Autodesk Inventor part; units mm, degrees
(part 14 of 18)
  line L295 (-10.395, -13.6654) -> (-10.3935, -13.6958)
  line L296 (9.9244, -17.7186) -> (9.9274, -17.7184)
  line L297 (10.1429, -17.706) -> (10.2016, -17.7027)
  line L298 (10.0945, -17.6651) -> (10.2016, -17.7027)
  line L299 (10.0388, -17.6683) -> (10.0945, -17.6651)
  line L300 (10.2016, -17.7027) -> (10.2019, -17.698)
  line L301 (10.0945, -17.6651) -> (10.0974, -17.6073)
  line L302 (10.1899, -15.782) -> (10.1905, -15.7701)
  line L303 (10.5029, -17.7271) -> (10.5027, -17.7312)
  line L304 (10.6831, -17.7208) -> (10.5027, -17.7312)
  line L305 (10.684, -17.7017) -> (10.6831, -17.7208)
  line L306 (10.5027, -17.7312) -> (10.9975, -17.9047)
  line L307 (11.1778, -17.8943) -> (10.9975, -17.9047)
  line L308 (10.6831, -17.7208) -> (11.1778, -17.8943)
  line L309 (11.1778, -17.8943) -> (11.1805, -17.8415)
  line L310 (11.0279, -17.9924) -> (10.9208, -17.9548)
  line L311 (11.0304, -17.9434) -> (11.0279, -17.9924)
  line L312 (10.9208, -17.9548) -> (10.6544, -17.9701)
  line L313 (11.0279, -17.9924) -> (10.6522, -18.014)
  line L314 (-10.131, -17.7025) -> (-10.0641, -17.6809)
  line L315 (-10.2521, -17.6674) -> (-10.0641, -17.6809)
  line L316 (-10.3599, -17.7021) -> (-10.2521, -17.6674)
  line L317 (-10.0641, -17.6809) -> (-10.0644, -17.6303)
  line L318 (-10.0765, -15.7777) -> (-10.0792, -15.3552)
  line L319 (-10.2521, -17.6674) -> (-10.2524, -17.6239)
  line L320 (-10.2645, -15.7689) -> (-10.2646, -15.7629)
  line L321 (-10.2782, -13.6655) -> (-10.2784, -13.6388)
  line L322 (9.0029, -17.7241) -> (9.7279, -17.6637)
  line L323 (9.6237, -17.6343) -> (9.7279, -17.6637)
  line L324 (9.3477, -17.6573) -> (9.6237, -17.6343)
  line L325 (9.7279, -17.6637) -> (9.728, -17.6538)
  line L326 (9.6237, -17.6343) -> (9.6238, -17.6121)
  line L327 (9.6503, -13.6367) -> (9.6506, -13.6057)
  line L328 (-7.4275, 0.4913) -> (-8.4227, 0.5954)
  line L329 (-11.2211, 1.3907) -> (-8.3706, 1.0926)
  ellipse E238 centre (-9.068, 1.1652) end of major axis (-11.5544, 1.4256) minor radius 0.0002 (-11.2211, 1.3907) -> (-11.5544, 1.4256) ccw
  line L330 (-11.7521, -0.4624) -> (-11.5544, 1.4256)
  line L331 (8.4338, 0.5941) -> (7.4385, 0.4902)
  line L332 (8.3818, 1.0914) -> (11.2323, 1.389)
  ellipse E239 centre (9.0792, 1.1638) end of major axis (11.5656, 1.4238) minor radius 0.0002 (11.5656, 1.4238) -> (11.2323, 1.389) ccw
  line L333 (11.5656, 1.4238) -> (11.763, -0.4642)
  ellipse E240 centre (-8.7944, -3.3251) end of major axis (-9.0427, -3.2961) minor radius 0
  ellipse E241 centre (-7.7259, -3.45) end of major axis (-8.3188, -3.3807) minor radius 0 (-8.2679, -3.3867) -> (-8.2679, -3.3867) ccw
  ellipse E242 centre (-11.2149, -3.0423) end of major axis (-10.4244, -3.1347) minor radius 0 (-11.5644, -3.0014) -> (-11.5645, -3.0015) ccw
  line L334 (-8.2679, -3.3865) -> (-12.108, -2.9378)
  ellipse E243 centre (-9.9578, -3.1893) end of major axis (-12.4408, -2.899) minor radius 0.0001 (-12.1007, -2.9387) -> (-12.4408, -2.899) ccw
  line L335 (-11.8177, -0.4547) -> (-8.9714, -0.7873)
  ellipse E244 centre (-9.6674, -0.7062) end of major axis (-12.1505, -0.4159) minor radius 0.0001 (-11.8177, -0.4547) -> (-12.1505, -0.4159) ccw
  line L336 (-12.4408, -2.899) -> (-12.1505, -0.4159)
  ellipse E245 centre (-4.296, -3.8511) end of major axis (-12.7385, -2.8641) minor radius 0.0004 (-12.3168, -2.9135) -> (-11.5646, -3.0016) ccw
  line L337 (-8.0358, -1.4) -> (-9.0294, -1.2839)
  ellipse E246 centre (8.8048, -3.3264) end of major axis (8.5565, -3.3554) minor radius 0
  ellipse E247 centre (7.7364, -3.4512) end of major axis (8.3292, -3.382) minor radius 0 (8.2784, -3.3879) -> (8.2784, -3.3879) ccw
  ellipse E248 centre (4.3063, -3.8518) end of major axis (12.749, -2.866) minor radius 0.0004 (11.5752, -3.0033) -> (12.3274, -2.9154) ccw
  ellipse E249 centre (9.9682, -3.1908) end of major axis (12.4514, -2.9009) minor radius 0.0001 (12.3274, -2.9154) -> (12.1186, -2.9397) ccw
  line L338 (12.1186, -2.9397) -> (8.2784, -3.3877)
  line L339 (8.9822, -0.7886) -> (11.8286, -0.4565)
  ellipse E250 centre (9.6783, -0.7077) end of major axis (12.1614, -0.4178) minor radius 0.0001 (12.1614, -0.4178) -> (11.8286, -0.4565) ccw
  line L340 (12.1614, -0.4178) -> (12.4514, -2.9009)
  ellipse E251 centre (11.2254, -3.044) end of major axis (10.4349, -3.1363) minor radius 0 (11.575, -3.0032) -> (11.5749, -3.0032) ccw
  line L341 (9.0402, -1.2853) -> (8.0466, -1.4012)
  line L342 (-6.9274, 2.4067) -> (-7.9232, 2.5012)
  line L343 (-10.7288, 3.2695) -> (-7.876, 2.999)
  ellipse E252 centre (-8.5735, 3.0651) end of major axis (-11.0623, 3.3012) minor radius 0 (-10.7288, 3.2695) -> (-11.0623, 3.3012) ccw
  line L344 (-11.2433, 1.3931) -> (-11.0623, 3.3012)
  line L345 (4.0938, 2.5867) -> (4.0057, 2.6011)
  line L346 (-3.9943, 2.6018) -> (-4.0824, 2.5874)
  line L347 (-5.7789, 2.8081) -> (-4.9943, 2.9362)
  line L348 (5.0057, 2.9355) -> (5.7903, 2.8072)
  line L349 (7.9346, 2.5) -> (6.9387, 2.4057)
  line L350 (7.8874, 2.9978) -> (10.7403, 3.2679)
  ellipse E253 centre (8.5849, 3.0638) end of major axis (11.0738, 3.2995) minor radius 0 (11.0738, 3.2995) -> (10.7403, 3.2679) ccw
  line L351 (11.0738, 3.2995) -> (11.2545, 1.3914)
  spline S0 degree 3 poles (-6.2703, 3.3864) (-6.2254, 3.4062) (-6.1365, 3.4454) (-6.0037, 3.5016) (-5.8729, 3.5551) (-5.7026, 3.622) (-5.494, 3.6996) (-5.3264, 3.7547) (-5.2441, 3.7817) knots 0 0 0 0 0.13379 0.264806 0.393183 0.519054 0.763783 1 1 1 1
  line L352 (-6.3254, 2.8599) -> (-6.2703, 3.3864)
  spline S1 degree 3 poles (-7.398, 3.7442) (-7.4114, 3.7431) (-7.4379, 3.741) (-7.477, 3.7389) (-7.5148, 3.7377) (-7.5511, 3.7377) (-7.5857, 3.7387) (-7.6185, 3.7408) (-7.6494, 3.744) (-7.6783, 3.7482) (-7.7052, 3.7533) (-7.7301, 3.7594) (-7.7528, 3.7663) (-7.7735, 3.774) (-7.7922, 3.7826) (-7.8092, 3.7922) (-7.8246, 3.8026) (-7.8337, 3.8106) (-7.8382, 3.8146) knots 0 0 0 0 0.088475 0.174424 0.25743 0.337089 0.413015 0.484966 0.552919 0.616878 0.676853 0.732867 0.784956 0.833184 0.87778 0.920162 0.960829 1 1 1 1
  ellipse E254 centre (-3.1382, 3.0582) end of major axis (-8.5695, 3.6268) minor radius 0.0004 (-6.2703, 3.3864) -> (-8.5695, 3.6268) ccw
  line L353 (-8.2557, 3.8812) -> (-8.5695, 3.6268)
  line L354 (-8.6278, 3.0703) -> (-8.5695, 3.6268)
  spline S2 degree 3 poles (-3.1442, 3.5227) (-3.1016, 3.547) (-3.0173, 3.5949) (-2.891, 3.6642) (-2.7665, 3.7307) (-2.6041, 3.8145) (-2.4047, 3.9129) (-2.2437, 3.9847) (-2.1647, 4.0199) knots 0 0 0 0 0.133763 0.26476 0.393126 0.518994 0.763738 1 1 1 1
  line L355 (-3.1442, 3.341) -> (-3.1442, 3.5227)
  line L356 (3.1557, 3.5222) -> (3.1557, 3.3405)
  spline S3 degree 3 poles (2.1763, 4.0196) (2.2553, 3.9843) (2.4162, 3.9125) (2.6156, 3.8141) (2.7781, 3.7302) (2.9026, 3.6638) (3.0288, 3.5945) (3.1131, 3.5465) (3.1557, 3.5222) knots 0 0 0 0 0.236262 0.481006 0.606874 0.73524 0.866237 1 1 1 1
  line L357 (-2.1647, 4.0199) -> (2.1763, 4.0196)
  ellipse E255 centre (0.0058, 3.5555) end of major axis (-4.9552, 3.5559) minor radius 0.5163 (2.6804, 3.9901) -> (2.1763, 4.0196) ccw
  ellipse E256 centre (0.0058, 3.5555) end of major axis (-4.9552, 3.5559) minor radius 0.5163 (-2.1647, 4.0199) -> (-2.6688, 3.9905) ccw
  ellipse E257 centre (0.0057, 3.0582) end of major axis (5.4667, 3.0578) minor radius 0.5683 (5.3031, 3.1959) -> (3.1557, 3.5222) ccw
  ellipse E258 centre (0.0057, 3.0582) end of major axis (-5.4553, 3.0586) minor radius 0.5683 (-3.1442, 3.5227) -> (-5.2916, 3.1967) ccw
  line L358 (6.2817, 3.3855) -> (6.3368, 2.859)
  spline S4 degree 3 poles (5.2556, 3.7809) (5.3379, 3.7538) (5.5055, 3.6987) (5.7141, 3.6211) (5.8844, 3.5542) (6.0152, 3.5007) (6.148, 3.4445) (6.2369, 3.4053) (6.2817, 3.3855) knots 0 0 0 0 0.236217 0.480946 0.606817 0.735194 0.86621 1 1 1 1
  spline S5 degree 3 poles (7.8493, 3.8136) (7.8447, 3.8096) (7.8351, 3.8013) (7.8189, 3.7906) (7.8009, 3.7807) (7.7812, 3.7719) (7.7597, 3.7639) (7.7365, 3.757) (7.7115, 3.751) (7.6849, 3.7461) (7.6565, 3.7422) (7.6263, 3.7393) (7.5943, 3.7375) (7.5606, 3.7366) (7.525, 3.7368) (7.4878, 3.738) (7.449, 3.7401) (7.4226, 3.7422) (7.4091, 3.7433) knots 0 0 0 0 0.040391 0.082789 0.1275 0.174786 0.22486 0.277901 0.334055 0.393442 0.45616 0.522411 0.592561 0.666584 0.744418 0.825989 0.911213 1 1 1 1
  ellipse E259 centre (3.1496, 3.0577) end of major axis (8.581, 3.6255) minor radius 0.0004 (8.581, 3.6255) -> (6.2817, 3.3855) ccw
  line L359 (8.2673, 3.8799) -> (8.581, 3.6255)
  line L360 (8.6392, 3.0689) -> (8.581, 3.6255)
  spline S6 degree 3 poles (-5.7981, 5.3131) (-5.7534, 5.3333) (-5.6649, 5.3734) (-5.5327, 5.4308) (-5.4024, 5.4856) (-5.2327, 5.5541) (-5.0249, 5.6338) (-4.8578, 5.6905) (-4.7758, 5.7183) knots 0 0 0 0 0.13379 0.264806 0.393183 0.519054 0.763783 1 1 1 1
  line L361 (-5.9686, 3.5159) -> (-5.7981, 5.3131)
  line L362 (-4.7758, 5.7183) -> (-3.9801, 5.6429)
  ellipse E260 centre (-2.6153, 5.5133) end of major axis (-7.5542, 5.9819) minor radius 0.0001 (-7.3844, 5.9658) -> (-7.5542, 5.9819) ccw
  ellipse E261 centre (-2.6153, 5.5133) end of major axis (-7.5542, 5.9819) minor radius 0.0001 (-4.7758, 5.7183) -> (-6.1112, 5.845) ccw
  spline S7 degree 3 poles (-6.1112, 5.845) (-6.1628, 5.8292) (-6.2638, 5.7981) (-6.4132, 5.7573) (-6.5562, 5.7223) (-6.692, 5.6938) (-6.8208, 5.672) (-6.9424, 5.6575) (-7.0389, 5.6518) (-7.1106, 5.6521) (-7.1588, 5.6549) (-7.2029, 5.66) (-7.2426, 5.6672) (-7.2779, 5.6764) (-7.3174, 5.6905) (-7.3588, 5.7133) (-7.3959, 5.7512) (-7.4169, 5.7986) (-7.4195, 5.8521) (-7.4083, 5.9091) (-7.3926, 5.9463) (-7.3844, 5.9658) knots 0 0 0 0 0.104135 0.203976 0.298889 0.388275 0.471711 0.551067 0.624597 0.658204 0.689291 0.717816 0.743784 0.767218 0.788166 0.824633 0.857384 0.888881 0.922221 0.959245 1 1 1 1
  ellipse E262 centre (-2.6626, 5.0156) end of major axis (-8.0992, 5.5313) minor radius 0.0001 (-5.7981, 5.3131) -> (-8.0992, 5.5313) ccw
  line L363 (-7.5542, 5.9819) -> (-8.0992, 5.5313)
  ellipse E263 centre (-6.0533, 5.8395) end of major axis (-4.5488, 5.6968) minor radius 0 (-7.3848, 5.9658) -> (-6.194, 5.8528) ccw
  line L364 (-8.2557, 3.8812) -> (-8.0992, 5.5313)
  spline S8 degree 3 poles (-3.144, 5.4364) (-3.1014, 5.4606) (-3.0171, 5.5087) (-2.8909, 5.578) (-2.7664, 5.6445) (-2.6039, 5.7284) (-2.4045, 5.8269) (-2.2436, 5.8988) (-2.1645, 5.9341) knots 0 0 0 0 0.133768 0.264768 0.393136 0.519004 0.763746 1 1 1 1
  line L365 (-3.1442, 3.7223) -> (-3.144, 5.4364)
  line L366 (3.1558, 5.4359) -> (3.1557, 3.7218)
  spline S9 degree 3 poles (2.1764, 5.9337) (2.2555, 5.8984) (2.4164, 5.8265) (2.6158, 5.728) (2.7782, 5.6441) (2.9027, 5.5776) (3.0289, 5.5082) (3.1132, 5.4602) (3.1558, 5.4359) knots 0 0 0 0 0.236254 0.480996 0.606864 0.735232 0.866232 1 1 1 1
  line L367 (-2.1645, 5.9341) -> (2.1764, 5.9337)
  ellipse E264 centre (0.0059, 5.5131) end of major axis (-4.9551, 5.5135) minor radius 0.4679 (3.5178, 5.8434) -> (2.1764, 5.9337) ccw
  ellipse E265 centre (0.0059, 5.5131) end of major axis (-4.9551, 5.5135) minor radius 0.4679 (-2.1645, 5.9341) -> (-3.5059, 5.8439) ccw
  spline S10 degree 3 poles (-3.5059, 5.8439) (-3.546, 5.8257) (-3.625, 5.7899) (-3.7424, 5.739) (-3.8563, 5.6915) (-3.9663, 5.6478) (-4.0719, 5.6081) (-4.1733, 5.5723) (-4.2708, 5.5406) (-4.364, 5.5134) (-4.451, 5.4913) (-4.5297, 5.4754) (-4.5985, 5.4659) (-4.6566, 5.4624) (-4.7048, 5.4646) (-4.7435, 5.473) (-4.775, 5.4866) (-4.7885, 5.5022) (-4.7948, 5.5095) knots 0 0 0 0 0.096483 0.190064 0.280343 0.366935 0.449463 0.527566 0.602572 0.674179 0.740358 0.79923 0.84998 0.89243 0.926709 0.955226 0.979191 1 1 1 1
  spline S11 degree 3 poles (4.8066, 5.5087) (4.8005, 5.5017) (4.7872, 5.4864) (4.756, 5.4729) (4.7173, 5.4645) (4.6697, 5.4619) (4.6138, 5.4648) (4.5492, 5.4734) (4.476, 5.4878) (4.3943, 5.5079) (4.3045, 5.5334) (4.2075, 5.5643) (4.1038, 5.6002) (3.9944, 5.6409) (3.88, 5.6861) (3.7198, 5.7525) (3.5992, 5.8067) (3.5178, 5.8434) knots 0 0 0 0 0.020314 0.043937 0.072556 0.107061 0.147904 0.195304 0.249736 0.311344 0.379674 0.454238 0.534533 0.62004 0.710199 0.804177 1 1 1 1
  ellipse E266 centre (0.0059, 5.0153) end of major axis (5.4669, 5.0149) minor radius 0.5151 (5.1609, 5.185) -> (3.1558, 5.4359) ccw
  ellipse E267 centre (0.0059, 5.0153) end of major axis (-5.4551, 5.0158) minor radius 0.5151 (-3.144, 5.4364) -> (-5.1492, 5.1857) ccw
  line L368 (5.8099, 5.3122) -> (5.9801, 3.515)
  spline S12 degree 3 poles (4.7876, 5.7176) (4.8697, 5.6898) (5.0367, 5.633) (5.2446, 5.5533) (5.4142, 5.4848) (5.5445, 5.43) (5.6767, 5.3725) (5.7652, 5.3324) (5.8099, 5.3122) knots 0 0 0 0 0.236217 0.480946 0.606817 0.735194 0.86621 1 1 1 1
  line L369 (3.9919, 5.6422) -> (4.7876, 5.7176)
  ellipse E268 centre (2.6271, 5.5129) end of major axis (-2.3117, 5.0452) minor radius 0.0001 (6.1245, 5.8442) -> (4.7895, 5.7178) ccw
  ellipse E269 centre (2.6271, 5.5129) end of major axis (7.566, 5.9807) minor radius 0.0001 (7.566, 5.9807) -> (7.3962, 5.9646) ccw
  spline S13 degree 3 poles (7.3963, 5.9646) (7.4047, 5.9446) (7.4206, 5.9071) (7.4315, 5.85) (7.4286, 5.7975) (7.4082, 5.7511) (7.3712, 5.7135) (7.3197, 5.6848) (7.2544, 5.6647) (7.1751, 5.6529) (7.0818, 5.6498) (6.9749, 5.6549) (6.8553, 5.668) (6.7244, 5.689) (6.5837, 5.7176) (6.435, 5.7537) (6.2803, 5.7958) (6.176, 5.8278) (6.1231, 5.8441) knots 0 0 0 0 0.041849 0.07857 0.111147 0.141904 0.174268 0.211184 0.254599 0.305659 0.365519 0.434561 0.512207 0.59776 0.690456 0.789354 0.89303 1 1 1 1
  ellipse E270 centre (2.6743, 5.0152) end of major axis (8.111, 5.5301) minor radius 0.0001 (8.111, 5.5301) -> (5.8099, 5.3122) ccw
  line L370 (7.566, 5.9807) -> (8.111, 5.5301)
  line L371 (8.2673, 3.8799) -> (8.111, 5.5301)
  ellipse E271 centre (-2.8258, 6.0418) end of major axis (-6.7195, 6.4495) minor radius 0.0003 (-3.1855, 6.0798) -> (-4.4498, 6.2121) ccw
  ellipse E272 centre (-4.7647, 6.2451) end of major axis (-4.5658, 6.2242) minor radius 0 (-4.6559, 6.2337) -> (-4.5658, 6.2242) ccw
  line L372 (-4.5657, 6.2243) -> (-4.5658, 6.2242)
  ellipse E273 centre (-4.3668, 6.2034) end of major axis (-4.5657, 6.2243) minor radius 0 (-4.4498, 6.2121) -> (-4.5657, 6.2243) ccw
  ellipse E274 centre (-2.8258, 6.0418) end of major axis (-6.1725, 6.3923) minor radius 0.0002 (-4.6559, 6.2337) -> (-6.1725, 6.3923) ccw
  line L373 (-6.1725, 6.3923) -> (-6.2286, 5.8561)
  ellipse E275 centre (-1.1805, 21.7559) end of major axis (-3.4282, 21.9913) minor radius 0.0002 (-3.154, 21.9627) -> (-3.4282, 21.9913) ccw
  line L374 (-3.4282, 21.9913) -> (-3.7247, 20.0442)
  line L375 (1.7559, 5.9338) -> (1.756, 6.3932)
  ellipse E276 centre (1.556, 6.3932) end of major axis (1.756, 6.3932) minor radius 0.0208 (1.756, 6.3932) -> (1.6394, 6.4121) ccw
  ellipse E277 centre (0.0059, 6.0419) end of major axis (-3.9091, 6.0422) minor radius 0.4074 (1.6394, 6.4121) -> (-1.6275, 6.4123) ccw
  ellipse E278 centre (1.956, 6.3524) end of major axis (1.756, 6.3524) minor radius 0.0208 (1.756, 6.3524) -> (1.8466, 6.335) ccw
  ellipse E279 centre (-1.944, 6.3527) end of major axis (-1.744, 6.3526) minor radius 0.0208 (-1.8346, 6.3352) -> (-1.744, 6.3526) ccw
  ellipse E280 centre (-1.544, 6.3934) end of major axis (-1.744, 6.3934) minor radius 0.0208 (-1.6275, 6.4123) -> (-1.744, 6.3934) ccw
  line L376 (-1.744, 6.3934) -> (-1.7441, 5.934)
  ellipse E281 centre (0.0059, 6.0419) end of major axis (3.3709, 6.0417) minor radius 0.3502 (3.3338, 6.0936) -> (1.8466, 6.335) ccw
  ellipse E282 centre (0.0059, 6.0419) end of major axis (-3.3591, 6.0422) minor radius 0.3502 (-1.8346, 6.3352) -> (-3.3219, 6.0941) ccw
  ellipse E283 centre (0.0071, 21.7561) end of major axis (2.2671, 21.756) minor radius 0.2352 (1.0452, 21.965) -> (-1.0309, 21.9651) ccw
  ellipse E284 centre (4.3787, 6.2028) end of major axis (4.5776, 6.2236) minor radius 0 (4.5776, 6.2236) -> (4.4617, 6.2115) ccw
  ellipse E285 centre (2.8377, 6.0414) end of major axis (-1.0561, 5.6343) minor radius 0.0003 (4.4617, 6.2115) -> (3.1974, 6.0793) ccw
  line L377 (4.5777, 6.2235) -> (4.5776, 6.2236)
  ellipse E286 centre (4.7766, 6.2443) end of major axis (4.5777, 6.2235) minor radius 0 (4.5777, 6.2235) -> (4.6678, 6.233) ccw
  ellipse E287 centre (2.8377, 6.0414) end of major axis (6.1844, 6.3913) minor radius 0.0002 (6.1844, 6.3913) -> (4.6678, 6.233) ccw
  line L378 (6.1844, 6.3913) -> (6.2405, 5.8552)
  ellipse E288 centre (1.1948, 21.7558) end of major axis (3.4425, 21.9908) minor radius 0.0002 (3.4425, 21.9908) -> (3.1684, 21.9622) ccw
  line L379 (3.4425, 21.9908) -> (3.7387, 20.0436)
  ellipse E289 centre (-1.5322, 19.7878) end of major axis (-3.7769, 20.0503) minor radius 0.0001 (-3.0188, 19.9617) -> (-3.7769, 20.0503) ccw
  line L380 (-3.7769, 20.0503) -> (-5.7087, 8.318)
  line L381 (-5.7576, 8.0211) -> (-6.0282, 6.3772)
  ellipse E290 centre (0.0058, 4.0949) end of major axis (-3.9092, 4.0952) minor radius 0.4538 (0.7242, 4.541) -> (0.6204, 4.5431) ccw
  ellipse E291 centre (0.0058, 4.0949) end of major axis (-3.9092, 4.0952) minor radius 0.4538 (0.3465, 4.547) -> (-0.3898, 4.5465) ccw
  ellipse E292 centre (0.0058, 4.0949) end of major axis (-3.9092, 4.0952) minor radius 0.4538 (-0.6087, 4.5432) -> (-0.7125, 4.5411) ccw
  ellipse E293 centre (0.007, 19.7884) end of major axis (2.267, 19.7882) minor radius 0.262 (1.716, 19.9597) -> (-1.702, 19.96) ccw
  ellipse E294 centre (1.5462, 19.7876) end of major axis (3.791, 20.0497) minor radius 0.0001 (3.791, 20.0497) -> (3.0328, 19.9613) ccw
  line L382 (3.791, 20.0497) -> (5.7209, 8.3171)
  line L383 (5.7697, 8.0202) -> (6.0402, 6.3763)
  ellipse E295 centre (-0.7937, 24.7162) end of major axis (-0.5896, 24.6969) minor radius 0 (-0.5896, 24.6969) -> (-0.8355, 24.7202) ccw
  ellipse E296 centre (-0.8349, 24.2822) end of major axis (-2.0644, 24.3988) minor radius 0 (-1.1783, 24.3148) -> (-2.0644, 24.3988) ccw
  line L384 (-2.0644, 24.3988) -> (-2.1166, 23.8482)
  arc A0 (-1.1612, 24.7267) -> (-2.0644, 24.3988) centre (-0.9749, 22.8057) ccw
  arc A1 (-0.4838, 24.6722) -> (-0.5896, 24.6969) centre (-0.9749, 22.8057) ccw
  ellipse E297 centre (-2.3792, 8.0022) end of major axis (-6.2767, 8.3719) minor radius 0 (-3.0173, 8.0627) -> (-4.0051, 8.1564) ccw
  ellipse E298 centre (-2.4737, 7.0066) end of major axis (-6.3712, 7.3764) minor radius 0 (-2.7241, 7.0304) -> (-4.0996, 7.1609) ccw
  line L385 (-4.1212, 8.1674) -> (-4.1212, 8.1674)
  line L386 (-4.2156, 7.1719) -> (-4.2156, 7.1719)
  ellipse E299 centre (-2.3792, 8.0022) end of major axis (-5.7292, 8.32) minor radius 0 (-4.2114, 8.176) -> (-5.7292, 8.32) ccw
  ellipse E300 centre (-2.4737, 7.0066) end of major axis (-5.8236, 7.3244) minor radius 0 (-4.3059, 7.1805) -> (-5.5824, 7.3016) ccw
  line L387 (-5.7292, 8.32) -> (-5.7576, 8.0211)
  ellipse E301 centre (-0.8871, 23.7316) end of major axis (-3.137, 23.945) minor radius 0 (-1.972, 23.8345) -> (-3.137, 23.945) ccw
  line L388 (-3.137, 23.945) -> (-3.4153, 21.99)
  ellipse E302 centre (0.0073, 24.2822) end of major axis (1.2423, 24.2821) minor radius 0.1165 (1.193, 24.3147) -> (-1.1783, 24.3149) ccw
  arc A2 (-0.1968, 24.7249) -> (-0.9743, 24.4674) centre (0.0072, 22.8057) ccw
  arc A3 (0.989, 24.4673) -> (0.2115, 24.7248) centre (0.0072, 22.8057) ccw
  ellipse E303 centre (1.556, 7.3248) end of major axis (1.756, 7.3248) minor radius 0.0189 (1.756, 7.3248) -> (1.6395, 7.3419) ccw
  line L389 (1.756, 7.3248) -> (1.7561, 8.3203)
  ellipse E304 centre (1.5561, 8.3203) end of major axis (1.7561, 8.3203) minor radius 0.0189 (1.7561, 8.3203) -> (1.6396, 8.3375) ccw
  ellipse E305 centre (0.0061, 8.002) end of major axis (-3.9089, 8.0023) minor radius 0.3693 (1.6396, 8.3375) -> (-1.6273, 8.3377) ccw
  ellipse E306 centre (0.006, 7.0064) end of major axis (-3.909, 7.0067) minor radius 0.3693 (1.6395, 7.3419) -> (-1.6274, 7.3422) ccw
  ellipse E307 centre (1.9561, 8.2833) end of major axis (1.7561, 8.2833) minor radius 0.0189 (1.7561, 8.2833) -> (1.8467, 8.2675) ccw
  ellipse E308 centre (-1.9439, 8.2836) end of major axis (-1.7439, 8.2836) minor radius 0.0189 (-1.8345, 8.2678) -> (-1.7439, 8.2836) ccw
  ellipse E309 centre (-1.5439, 8.3206) end of major axis (-1.7439, 8.3206) minor radius 0.0189 (-1.6273, 8.3377) -> (-1.7439, 8.3206) ccw
  ellipse E310 centre (-1.544, 7.325) end of major axis (-1.744, 7.325) minor radius 0.0189 (-1.6274, 7.3422) -> (-1.744, 7.325) ccw
  line L390 (-1.7439, 8.3206) -> (-1.744, 7.325)
  ellipse E311 centre (1.956, 7.2878) end of major axis (1.756, 7.2878) minor radius 0.0189 (1.756, 7.2878) -> (1.8466, 7.272) ccw
  line L391 (1.756, 7.2878) -> (1.756, 7.3248)
  ellipse E312 centre (-1.944, 7.2881) end of major axis (-1.744, 7.2881) minor radius 0.0189 (-1.8346, 7.2723) -> (-1.744, 7.2881) ccw
  line L392 (-1.744, 7.325) -> (-1.744, 7.2881)
  ellipse E313 centre (0.0061, 8.002) end of major axis (3.3711, 8.0017) minor radius 0.3174 (3.2567, 8.0838) -> (1.8467, 8.2675) ccw
  ellipse E314 centre (0.0061, 8.002) end of major axis (-3.3589, 8.0022) minor radius 0.3174 (-1.8345, 8.2678) -> (-3.2445, 8.0843) ccw
  ellipse E315 centre (0.006, 7.0064) end of major axis (-3.359, 7.0067) minor radius 0.3174 (-3.2638, 7.0816) -> (-3.3332, 7.0459) ccw
  ellipse E316 centre (0.006, 7.0064) end of major axis (3.371, 7.0062) minor radius 0.3174 (-1.8346, 7.2723) -> (-3.0548, 7.1385) ccw
  ellipse E317 centre (0.006, 7.0064) end of major axis (3.371, 7.0062) minor radius 0.3174 (3.0669, 7.1381) -> (1.8466, 7.272) ccw
  ellipse E318 centre (0.006, 7.0064) end of major axis (3.371, 7.0062) minor radius 0.3174 (3.3453, 7.0454) -> (3.2759, 7.0811) ccw
  ellipse E319 centre (0.0073, 23.7315) end of major axis (2.2673, 23.7314) minor radius 0.2132 (1.9869, 23.8342) -> (-1.9723, 23.8345) ccw
  ellipse E320 centre (0.8084, 24.7161) end of major axis (0.6043, 24.6968) minor radius 0 (0.8502, 24.7201) -> (0.6043, 24.6968) ccw
  ellipse E321 centre (0.8495, 24.2821) end of major axis (2.079, 24.3985) minor radius 0 (2.079, 24.3985) -> (1.193, 24.3146) ccw
  line L393 (2.079, 24.3985) -> (2.1312, 23.8479)
  arc A4 (0.6043, 24.6968) -> (0.4985, 24.6721) centre (0.9894, 22.8056) ccw
  arc A5 (2.079, 24.3985) -> (1.1759, 24.7265) centre (0.9894, 22.8056) ccw
  ellipse E322 centre (2.3914, 8.0018) end of major axis (-1.5061, 7.6327) minor radius 0 (4.0179, 8.1559) -> (3.0301, 8.0623) ccw
  ellipse E323 centre (2.4857, 7.0063) end of major axis (-1.4118, 6.6371) minor radius 0 (4.1121, 7.1603) -> (2.7367, 7.0301) ccw
  line L394 (4.1334, 8.1668) -> (4.1334, 8.1668)
  line L395 (4.2277, 7.1713) -> (4.2277, 7.1713)
  ellipse E324 centre (2.3914, 8.0018) end of major axis (5.7414, 8.3191) minor radius 0 (5.7414, 8.3191) -> (4.2235, 8.1754) ccw
  ellipse E325 centre (2.4857, 7.0063) end of major axis (5.8357, 7.3235) minor radius 0 (5.5945, 7.3007) -> (4.3179, 7.1798) ccw
  line L396 (5.7414, 8.3191) -> (5.7697, 8.0202)
  ellipse E326 centre (0.9017, 23.7314) end of major axis (3.1516, 23.9445) minor radius 0 (3.1516, 23.9445) -> (1.9866, 23.8342) ccw
  line L397 (3.1516, 23.9445) -> (3.4296, 21.9894)
  line L398 (7.1686, -28.47) -> (6.503, -26.7548)
  line L399 (9.2433, -28.4702) -> (8.7012, -26.5895)
  line L400 (-9.7907, -28.4687) -> (-9.8927, -26.4495)
  line L401 (-7.7204, -28.4689) -> (-7.6178, -26.5179)
  line L402 (7.1241, -27.8075) -> (6.891, -26.7073)
  line L403 (9.2552, -27.754) -> (9.1137, -26.4991)
  line L404 (-9.2484, -27.7526) -> (-9.1068, -26.4977)
  line L405 (-7.1174, -27.8064) -> (-6.8841, -26.7063)
  line L406 (7.7271, -28.47) -> (7.6247, -26.5191)
  line L407 (9.7974, -28.4702) -> (9.8986, -26.4701)
  line L408 (-9.2366, -28.4688) -> (-8.692, -26.5804)
  line L409 (-7.1619, -28.4689) -> (-6.4961, -26.7538)
  line L410 (7.4032, -27.0593) -> (7.3205, -26.6137)
  line L411 (9.5891, -27.074) -> (9.5284, -26.4528)
  line L412 (-9.5822, -27.0726) -> (-9.5215, -26.4513)
  line L413 (-7.3963, -27.0582) -> (-7.3136, -26.6126)
  ellipse E327 centre (-10.4185, -13.2181) end of major axis (-10.4918, -13.0429) minor radius 0.1721 (-10.5933, -13.21) -> (-10.4874, -13.3848) ccw
  ellipse E328 centre (-10.4771, -13.2427) end of major axis (-10.4038, -13.418) minor radius 0.1721 (-10.6124, -13.3509) -> (-10.5542, -13.4047) ccw
  ellipse E329 centre (-10.4073, -16.022) end of major axis (-10.4807, -15.8468) minor radius 0.1721 (-10.5195, -15.8702) -> (-10.5397, -15.8899) ccw
  ellipse E330 centre (-10.6685, -13.241) end of major axis (-10.6774, -13.4308) minor radius 0.074 (-10.6638, -13.4283) -> (-10.5942, -13.2099) ccw
  ellipse E331 centre (-10.8065, -13.2346) end of major axis (-10.8154, -13.4244) minor radius 0.074 (-10.8018, -13.4218) -> (-10.7322, -13.2035) ccw
  ellipse E332 centre (-10.7367, -16.0139) end of major axis (-10.7278, -15.8241) minor radius 0.074 (-10.6624, -15.9828) -> (-10.7414, -15.8266) ccw
  ellipse E333 centre (-10.3486, -15.9975) end of major axis (-10.422, -15.8222) minor radius 0.1721 (-10.4528, -15.8394) -> (-10.5234, -15.9893) ccw
  ellipse E334 centre (-10.5987, -16.0203) end of major axis (-10.5898, -15.8306) minor radius 0.074 (-10.5244, -15.9893) -> (-10.5898, -15.8306) ccw
  line L414 (-10.5898, -15.8306) -> (-10.7278, -15.8241)
  line L415 (-10.3145, -13.4373) -> (-10.4056, -13.4331)
  line L416 (-10.3317, -13.4092) -> (-10.2128, -13.4148)
  line L417 (-9.7276, -15.6797) -> (-9.7385, -15.2452)
  line L418 (-9.7737, -13.8461) -> (-9.7786, -13.6495)
  line L419 (-11.0395, -13.5213) -> (-10.8018, -13.4218)
  line L420 (-10.6638, -13.4283) -> (-10.7944, -13.483)
  line L421 (-10.7414, -15.8266) -> (-10.842, -15.8687)
  line L422 (-11.0628, -15.7719) -> (-11.1138, -13.7417)
  line L423 (-10.1457, -15.8199) -> (-10.2272, -15.8161)
  line L424 (-10.9758, -13.7481) -> (-10.9248, -15.7784)
  line L425 (-9.7199, -13.6249) -> (-9.7141, -13.8596)
  line L426 (-9.6882, -14.8878) -> (-9.6689, -15.6552)
  ellipse E335 centre (-10.5118, -11.8629) end of major axis (-10.5851, -11.6876) minor radius 0.1721 (-10.5851, -11.6876) -> (-10.6442, -11.7307) ccw
  ellipse E336 centre (-10.3726, -17.4018) end of major axis (-10.2993, -17.5771) minor radius 0.1721 (-10.508, -17.51) -> (-10.4962, -17.5248) ccw
  ellipse E337 centre (-10.314, -17.3773) end of major axis (-10.3873, -17.202) minor radius 0.1721 (-10.4888, -17.3691) -> (-10.4293, -17.5091) ccw
  ellipse E338 centre (-10.4531, -11.8383) end of major axis (-10.5265, -11.6631) minor radius 0.1721 (-10.5117, -11.6577) -> (-10.6279, -11.8302) ccw
  line L427 (-10.5851, -11.6876) -> (-10.5265, -11.6631)
  line L428 (-10.3462, -17.5901) -> (-9.333, -17.6375)
  line L429 (-10.4888, -17.3691) -> (-10.5234, -15.9893)
  line L430 (-9.9216, -17.5827) -> (-10.2724, -17.5663)
  line L431 (-10.244, -11.6611) -> (-10.1954, -11.6634)
  line L432 (-10.5933, -13.21) -> (-10.6279, -11.8302)
  ellipse E339 centre (-9.9024, -15.6716) end of major axis (-9.8291, -15.8468) minor radius 0.1721 (-9.7624, -15.7942) -> (-9.7276, -15.6797) ccw
  ellipse E340 centre (-9.9534, -13.6413) end of major axis (-9.8801, -13.8165) minor radius 0.1721 (-9.7786, -13.6495) -> (-9.7866, -13.5977) ccw
  ellipse E341 centre (-10.9885, -15.7408) end of major axis (-10.9974, -15.9306) minor radius 0.074 (-11.0628, -15.7719) -> (-11.0467, -15.8737) ccw
  ellipse E342 centre (-11.0395, -13.7106) end of major axis (-11.0307, -13.5208) minor radius 0.074 (-11.0571, -13.5316) -> (-11.1138, -13.7417) ccw
  ellipse E343 centre (-9.8948, -13.6167) end of major axis (-9.9681, -13.4415) minor radius 0.1721 (-9.7199, -13.6249) -> (-9.748, -13.5262) ccw
  ellipse E344 centre (-9.8438, -15.647) end of major axis (-9.7704, -15.8223) minor radius 0.1721 (-9.7286, -15.7964) -> (-9.6689, -15.6552) ccw
  ellipse E345 centre (-10.8505, -15.7473) end of major axis (-10.8417, -15.5575) minor radius 0.074 (-10.9248, -15.7784) -> (-10.9147, -15.8595) ccw
  ellipse E346 centre (-10.9015, -13.717) end of major axis (-10.8927, -13.5272) minor radius 0.074 (-10.9721, -13.6754) -> (-10.9758, -13.7481) ccw
  line L433 (-10.7322, -13.2035) -> (-10.7669, -11.8237)
  line L434 (-10.8459, -11.6675) -> (-11.0308, -11.7449)
  line L435 (-11.1442, -17.768) -> (-10.6973, -17.581)
  line L436 (-10.6277, -17.3626) -> (-10.6624, -15.9828)
  line L437 (-10.5942, -13.2099) -> (-10.6289, -11.8301)
  line L438 (-10.4897, -17.3691) -> (-10.5244, -15.9893)
  line L439 (-11.4118, -17.9442) -> (-10.5593, -17.5874)
  ellipse E347 centre (-10.8412, -11.8548) end of major axis (-10.8323, -11.665) minor radius 0.074 (-10.7669, -11.8237) -> (-10.8459, -11.6675) ccw
  ellipse E348 centre (-10.702, -17.3937) end of major axis (-10.7109, -17.5835) minor radius 0.074 (-10.6973, -17.581) -> (-10.6277, -17.3626) ccw
  ellipse E349 centre (-10.7032, -11.8612) end of major axis (-10.6943, -11.6714) minor radius 0.074 (-10.6289, -11.8301) -> (-10.6943, -11.6714) ccw
  ellipse E350 centre (-10.564, -17.4002) end of major axis (-10.5729, -17.5899) minor radius 0.074 (-10.5593, -17.5874) -> (-10.4897, -17.3691) ccw
  line L440 (-10.8323, -11.665) -> (-10.6943, -11.6714)
  line L441 (-10.6433, -18.0256) -> (-11.2796, -17.9959)
  line L442 (-11.3382, -18.0204) -> (-10.6419, -18.053)
  ellipse E351 centre (-11.1818, -17.955) end of major axis (-11.4317, -17.9612) minor radius 0.0419 (-11.4118, -17.9442) -> (-11.2796, -17.9959) ccw
  ellipse E352 centre (-11.1818, -17.955) end of major axis (-11.5817, -17.965) minor radius 0.067 (-11.5798, -17.9582) -> (-11.3382, -18.0204) ccw
  line L443 (-11.5818, -17.9591) -> (-11.5817, -17.965)
  line L444 (9.4455, -13.3827) -> (9.7264, -13.3723)
  line L445 (9.5775, -15.6222) -> (9.4446, -14.3526)
  ellipse E353 centre (9.6129, -11.7904) end of major axis (9.588, -11.6021) minor radius 0.1017 (9.6923, -11.695) -> (9.5932, -11.6016) ccw
  line L446 (9.5932, -11.6016) -> (9.4899, -11.6055)
  line L447 (9.6809, -17.5835) -> (9.9756, -17.5725)
  line L448 (9.9861, -17.5722) -> (10.0546, -17.5696)
  line L449 (9.4941, -17.6023) -> (9.6004, -17.5984)
  ellipse E354 centre (9.6794, -15.6184) end of major axis (9.7043, -15.8068) minor radius 0.1017 (9.5775, -15.6222) -> (9.667, -15.7993) ccw
  ellipse E355 centre (9.4652, -13.5715) end of major axis (9.4404, -13.3831) minor radius 0.1017 (9.4455, -13.3827) -> (9.4451, -13.3827) ccw
  line L450 (-9.3696, -11.6205) -> (-9.4596, -11.6203)
  line L451 (-9.7048, -17.5828) -> (-9.6652, -17.5829)
  line L452 (-9.4762, -17.5832) -> (-9.2454, -17.5836)
  line L453 (-9.1525, -17.3949) -> (-9.0798, -16.7016)
  line L454 (-9.5815, -17.5997) -> (-9.5124, -17.5998)
  ellipse E356 centre (-9.2256, -17.3948) end of major axis (-9.2487, -17.5834) minor radius 0.0727 (-9.2454, -17.5836) -> (-9.1525, -17.3949) ccw
  line L455 (-9.2142, -15.8146) -> (-9.2578, -15.8146)
  ellipse E357 centre (-9.0928, -11.6653) end of major axis (-9.4906, -11.6236) minor radius 0.0171 (-9.4596, -11.6203) -> (-9.4906, -11.6236) ccw
  line L456 (-9.4906, -11.6236) -> (-9.4911, -11.6285)
  line L457 (11.4179, -17.9448) -> (11.0286, -17.9774)
  line L458 (10.6509, -18.039) -> (11.4993, -17.9679)
  ellipse E358 centre (11.4226, -17.7575) end of major axis (11.3708, -17.9403) minor radius 0.1568 (11.4179, -17.9448) -> (11.5023, -17.9099) ccw
  ellipse E359 centre (11.5041, -17.7806) end of major axis (11.4523, -17.9634) minor radius 0.1568 (11.4993, -17.9679) -> (11.5861, -17.9311) ccw
  line L459 (10.6787, -11.6745) -> (10.6474, -11.6656)
  line L460 (10.4979, -17.5791) -> (10.9377, -17.7037)
  line L461 (10.4903, -17.6232) -> (11.5564, -17.9252)
  line L462 (10.603, -13.42) -> (10.9181, -13.5092)
  line L463 (11.0166, -13.7257) -> (10.9653, -15.756)
  ellipse E360 centre (10.2674, -13.4481) end of major axis (10.6672, -13.4582) minor radius 0.067 (10.603, -13.42) -> (10.3781, -13.3865) ccw
  line L464 (9.6449, -13.4205) -> (9.9853, -13.392)
  ellipse E361 centre (10.2674, -13.4481) end of major axis (10.0174, -13.4418) minor radius 0.0419 (10.2515, -13.406) -> (10.1375, -13.4092) ccw
  line L465 (10.6336, -13.4749) -> (10.5682, -13.4563)
  ellipse E362 centre (10.2066, -15.8529) end of major axis (9.8067, -15.8428) minor radius 0.067 (10.5324, -15.8221) -> (10.2569, -15.7877) ccw
  line L466 (9.5478, -13.6455) -> (9.5414, -13.8989)
  ellipse E363 centre (10.9134, -13.6965) end of major axis (10.8975, -13.5072) minor radius 0.1025 (11.0166, -13.7257) -> (10.9181, -13.5092) ccw
  ellipse E364 centre (10.8621, -15.7268) end of major axis (10.8462, -15.5374) minor radius 0.1025 (10.9374, -15.8709) -> (10.9653, -15.756) ccw
  ellipse E365 centre (9.7072, -13.6321) end of major axis (9.759, -13.4493) minor radius 0.1568 (9.559, -13.5808) -> (9.5478, -13.6455) ccw
  ellipse E366 centre (9.6257, -13.609) end of major axis (9.5739, -13.7918) minor radius 0.1568 (9.5907, -13.431) -> (9.4934, -13.5204) ccw
  line L467 (9.3392, -17.6264) -> (9.6361, -17.6015)
  line L468 (9.9681, -17.5737) -> (10.0264, -17.5688)
  ellipse E367 centre (10.1622, -17.6072) end of major axis (10.4122, -17.6136) minor radius 0.0419 (10.1714, -17.5656) -> (10.0264, -17.5688) ccw
  ellipse E368 centre (10.3117, -11.6938) end of major axis (9.9118, -11.6837) minor radius 0.067 (10.6474, -11.6656) -> (10.3438, -11.6278) ccw
  ellipse E369 centre (10.1622, -17.6072) end of major axis (9.7624, -17.5971) minor radius 0.067 (10.4979, -17.5791) -> (10.3333, -17.5509) ccw
  ellipse E370 centre (11.5611, -17.7379) end of major axis (11.577, -17.9273) minor radius 0.1025 (11.5564, -17.9252) -> (11.5756, -17.9274) ccw
  line L469 (9.0712, -17.9822) -> (9.0269, -17.9697)
  ellipse E371 centre (-10.7565, -13.2512) end of major axis (-10.8325, -13.077) minor radius 0.169 (-10.9287, -13.2453) -> (-10.8385, -13.4073) ccw
  ellipse E372 centre (-10.8193, -13.2786) end of major axis (-10.7433, -13.4527) minor radius 0.169 (-10.9475, -13.3912) -> (-10.897, -13.4376) ccw
  ellipse E373 centre (-11.0092, -13.28) end of major axis (-11.0157, -13.4699) minor radius 0.0799 (-10.9998, -13.4667) -> (-10.9296, -13.2453) ccw
  ellipse E374 centre (-11.1452, -13.2754) end of major axis (-11.1517, -13.4653) minor radius 0.0799 (-11.1358, -13.4621) -> (-11.0656, -13.2407) ccw
  ellipse E375 centre (-11.0053, -16.0465) end of major axis (-10.9989, -15.8566) minor radius 0.0799 (-10.9258, -16.0117) -> (-11.0148, -15.8598) ccw
  ellipse E376 centre (-10.6166, -16.0222) end of major axis (-10.6926, -15.8481) minor radius 0.169 (-10.7548, -15.898) -> (-10.7889, -16.0164) ccw
  ellipse E377 centre (-10.8693, -16.0511) end of major axis (-10.8629, -15.8612) minor radius 0.0799 (-10.7898, -16.0164) -> (-10.8629, -15.8612) ccw
  line L470 (-10.8629, -15.8612) -> (-10.9989, -15.8566)
  line L471 (-10.6797, -13.4697) -> (-10.7566, -13.4671)
  line L472 (-10.6912, -13.4398) -> (-10.6159, -13.4423)
  line L473 (-10.0192, -15.6993) -> (-10.0372, -15.3416)
  line L474 (-10.1117, -13.867) -> (-10.1213, -13.675)
  line L475 (-11.3955, -13.5755) -> (-11.1358, -13.4621)
  line L476 (-10.9998, -13.4667) -> (-11.2595, -13.5802)
  line L477 (-12.049, -13.8609) -> (-11.806, -13.7548)
  line L478 (-11.717, -13.9068) -> (-11.6148, -15.931)
  line L479 (-11.685, -16.1525) -> (-11.9279, -16.2586)
  line L480 (-11.0148, -15.8598) -> (-11.2745, -15.9732)
  line L481 (-11.3635, -15.8213) -> (-11.4657, -13.797)
  line L482 (-10.5408, -15.8384) -> (-10.5717, -15.8374)
  line L483 (-11.3297, -13.8016) -> (-11.2275, -15.8259)
  ellipse E378 centre (-11.6863, -13.8732) end of major axis (-12.0858, -13.8934) minor radius 0.0715 (-12.049, -13.8609) -> (-11.8538, -13.9464) ccw
  line L484 (-11.7148, -13.9511) -> (-11.8538, -13.9464)
  line L485 (-11.791, -13.9189) -> (-11.7333, -13.9209)
  ellipse E379 centre (-11.6863, -13.8732) end of major axis (-11.936, -13.8858) minor radius 0.0447 (-11.913, -13.8655) -> (-11.791, -13.9189) ccw
  line L486 (-11.7434, -13.7915) -> (-11.913, -13.8655)
  ellipse E380 centre (-11.5652, -16.2709) end of major axis (-11.9647, -16.291) minor radius 0.0715 (-11.9279, -16.2586) -> (-11.9647, -16.291) ccw
  line L487 (-10.0585, -13.6476) -> (-10.0442, -13.9309)
  line L488 (-9.974, -15.3212) -> (-9.9563, -15.6719)
  ellipse E381 centre (-10.8887, -11.9029) end of major axis (-10.9648, -11.7288) minor radius 0.169 (-10.9648, -11.7288) -> (-11.0189, -11.7687) ccw
  ellipse E382 centre (-10.61, -17.4254) end of major axis (-10.5339, -17.5995) minor radius 0.169 (-10.6154, -17.6109) -> (-10.6005, -17.6121) ccw
  ellipse E383 centre (-10.5471, -17.3979) end of major axis (-10.6232, -17.2238) minor radius 0.169 (-10.5521, -17.5835) -> (-10.5377, -17.5846) ccw
  ellipse E384 centre (-10.5471, -17.3979) end of major axis (-10.6232, -17.2238) minor radius 0.169 (-10.7194, -17.3921) -> (-10.7022, -17.4651) ccw
  ellipse E385 centre (-10.8259, -11.8755) end of major axis (-10.9019, -11.7013) minor radius 0.169 (-10.8958, -11.6988) -> (-10.9982, -11.8696) ccw
  line L489 (-10.9648, -11.7288) -> (-10.9019, -11.7013)
  line L490 (-10.6005, -17.6121) -> (-10.5839, -17.6126)
  line L491 (-10.432, -17.6178) -> (-9.3384, -17.6549)
  line L492 (-10.7194, -17.3921) -> (-10.7889, -16.0164)
  line L493 (-10.2665, -17.5938) -> (-10.3491, -17.591)
  line L494 (-10.5172, -17.5853) -> (-10.5377, -17.5846)
  line L495 (-10.661, -11.6947) -> (-10.6431, -11.6953)
  line L496 (-10.9287, -13.2453) -> (-10.9982, -11.8696)
  ellipse E386 centre (-10.1914, -15.6934) end of major axis (-10.1154, -15.8676) minor radius 0.169 (-10.0321, -15.7797) -> (-10.0192, -15.6993) ccw
  ellipse E387 centre (-10.2936, -13.6692) end of major axis (-10.2176, -13.8433) minor radius 0.169 (-10.1213, -13.675) -> (-10.1287, -13.6298) ccw
  ellipse E388 centre (-11.7966, -13.9415) end of major axis (-11.7901, -13.7516) minor radius 0.0799 (-11.717, -13.9068) -> (-11.806, -13.7548) ccw
  ellipse E389 centre (-11.6944, -15.9658) end of major axis (-11.7008, -16.1557) minor radius 0.0799 (-11.685, -16.1525) -> (-11.6148, -15.931) ccw
  ellipse E390 centre (-11.2839, -15.7865) end of major axis (-11.2903, -15.9764) minor radius 0.0799 (-11.3635, -15.8213) -> (-11.2745, -15.9732) ccw
  ellipse E391 centre (-11.3861, -13.7623) end of major axis (-11.3796, -13.5724) minor radius 0.0799 (-11.3955, -13.5755) -> (-11.4657, -13.797) ccw
  ellipse E392 centre (-10.2308, -13.6418) end of major axis (-10.3068, -13.4676) minor radius 0.169 (-10.0585, -13.6476) -> (-10.0644, -13.6081) ccw
  ellipse E393 centre (-10.1286, -15.666) end of major axis (-10.2046, -15.4919) minor radius 0.169 (-9.9907, -15.7907) -> (-9.9563, -15.6719) ccw
  ellipse E394 centre (-11.1479, -15.7911) end of major axis (-11.1415, -15.6012) minor radius 0.0799 (-11.2275, -15.8259) -> (-11.2011, -15.9412) ccw
  ellipse E395 centre (-11.2501, -13.7669) end of major axis (-11.2436, -13.577) minor radius 0.0799 (-11.2595, -13.5802) -> (-11.3297, -13.8016) ccw
  line L497 (-11.0656, -13.2407) -> (-11.1351, -11.865)
  line L498 (-11.2241, -11.713) -> (-12.1373, -12.1118)
  line L499 (-11.8396, -18.0077) -> (-10.9265, -17.6089)
  line L500 (-10.8563, -17.3875) -> (-10.9258, -16.0117)
  line L501 (-10.9296, -13.2453) -> (-10.9991, -11.8696)
  line L502 (-10.7203, -17.3921) -> (-10.7898, -16.0164)
  line L503 (-11.7036, -18.0123) -> (-10.7905, -17.6135)
  ellipse E396 centre (-11.2147, -11.8997) end of major axis (-11.2082, -11.7098) minor radius 0.0799 (-11.1351, -11.865) -> (-11.2241, -11.713) ccw
  ellipse E397 centre (-10.9359, -17.4222) end of major axis (-10.9423, -17.6121) minor radius 0.0799 (-10.9265, -17.6089) -> (-10.8563, -17.3875) ccw
  ellipse E398 centre (-11.0787, -11.9043) end of major axis (-11.0722, -11.7144) minor radius 0.0799 (-10.9991, -11.8696) -> (-11.0722, -11.7144) ccw
  ellipse E399 centre (-10.7999, -17.4268) end of major axis (-10.8063, -17.6167) minor radius 0.0799 (-10.7905, -17.6135) -> (-10.7203, -17.3921) ccw
  line L504 (-11.2082, -11.7098) -> (-11.0722, -11.7144)
  line L505 (-10.6397, -18.0976) -> (-11.5817, -18.0657)
  line L506 (-11.6445, -18.0931) -> (-10.6382, -18.1273)
  ellipse E400 centre (-11.4769, -18.02) end of major axis (-11.7266, -18.0326) minor radius 0.0447 (-11.7036, -18.0123) -> (-11.5817, -18.0657) ccw
  ellipse E401 centre (-11.7746, -12.1241) end of major axis (-12.1741, -12.1443) minor radius 0.0715 (-12.1373, -12.1118) -> (-12.1741, -12.1443) ccw
  ellipse E402 centre (-11.4769, -18.02) end of major axis (-11.8764, -18.0401) minor radius 0.0715 (-11.8396, -18.0077) -> (-11.6445, -18.0931) ccw
  line L507 (-12.1741, -12.1443) -> (-12.0858, -13.8934)
  line L508 (-11.9647, -16.291) -> (-11.8764, -18.0401)
  ellipse E403 centre (9.6218, -13.1675) end of major axis (9.6454, -13.356) minor radius 0.0959 (9.643, -13.3563) -> (9.7175, -13.1602) ccw
  line L509 (9.6454, -13.356) -> (9.6188, -13.3594)
  line L510 (9.4438, -13.3714) -> (9.643, -13.3563)
  line L511 (9.7998, -15.7892) -> (9.6038, -15.8041)
  line L512 (9.4868, -15.6226) -> (9.3867, -14.7345)
  line L513 (9.7175, -13.1602) -> (9.5608, -11.7693)
  line L514 (9.4437, -11.5879) -> (9.2374, -11.6035)
  line L515 (9.017, -17.6322) -> (9.9579, -17.5607)
  line L516 (8.9456, -17.644) -> (9.5765, -17.5961)
  ellipse E404 centre (9.465, -11.7766) end of major axis (9.4414, -11.5881) minor radius 0.0959 (9.5608, -11.7693) -> (9.4437, -11.5879) ccw
  ellipse E405 centre (9.5825, -15.6153) end of major axis (9.6062, -15.8039) minor radius 0.0959 (9.4868, -15.6226) -> (9.6038, -15.8041) ccw
  ellipse E406 centre (8.6745, -17.6752) end of major axis (8.277, -17.72) minor radius 0.0085 (9.017, -17.6322) -> (8.9464, -17.6383) ccw
  line L517 (-9.2286, -11.6057) -> (-9.3312, -11.599)
  line L518 (-9.8559, -17.5695) -> (-9.1037, -17.6189)
  line L519 (-9.0039, -17.4353) -> (-8.9889, -17.3021)
  line L520 (-9.5406, -17.5979) -> (-8.9681, -17.6355)
  line L521 (-9.5308, -13.3674) -> (-9.4353, -13.3736)
  line L522 (-9.3703, -14.7838) -> (-9.4651, -15.6235)
  line L523 (-9.5648, -15.8072) -> (-9.8044, -15.7914)
  ellipse E407 centre (-9.1693, -13.4117) end of major axis (-9.5667, -13.3669) minor radius 0.0085 (-9.5308, -13.3674) -> (-9.5579, -13.3661) ccw
  ellipse E408 centre (-9.4428, -15.8358) end of major axis (-9.8403, -15.7909) minor radius 0.0085 (-9.8044, -15.7914) -> (-9.8403, -15.7909) ccw
  ellipse E409 centre (-9.5435, -15.6184) end of major axis (-9.5667, -15.807) minor radius 0.0785 (-9.5648, -15.8072) -> (-9.4651, -15.6235) ccw
  ellipse E410 centre (-9.0824, -17.4301) end of major axis (-9.1055, -17.6187) minor radius 0.0785 (-9.1037, -17.6189) -> (-9.0039, -17.4353) ccw
  ellipse E411 centre (-8.9468, -17.4467) end of major axis (-8.9699, -17.6353) minor radius 0.0785 (-8.9681, -17.6355) -> (-8.9398, -17.6258) ccw
  ellipse E412 centre (-8.9697, -11.6434) end of major axis (-9.3672, -11.5985) minor radius 0.0085 (-9.3312, -11.599) -> (-9.3672, -11.5985) ccw
  line L524 (-9.3672, -11.5985) -> (-9.3703, -11.6261)
  line L525 (-9.8403, -15.7909) -> (-9.8415, -15.8014)
  ellipse E413 centre (11.975, -13.724) end of major axis (11.9121, -13.9033) minor radius 0.1599 (11.9656, -13.9107) -> (12.0631, -13.8697) ccw
  ellipse E414 centre (11.8985, -13.6972) end of major axis (11.8356, -13.8765) minor radius 0.1599 (11.8891, -13.8839) -> (11.9795, -13.8486) ccw
  ellipse E415 centre (12.0421, -13.6806) end of major axis (12.053, -13.8703) minor radius 0.0969 (12.0327, -13.8673) -> (12.053, -13.8703) ccw
  ellipse E416 centre (12.1709, -13.6732) end of major axis (12.1818, -13.8629) minor radius 0.0969 (12.1615, -13.8599) -> (12.2678, -13.7072) ccw
  ellipse E417 centre (12.0306, -16.4442) end of major axis (12.0197, -16.2546) minor radius 0.0969 (12.1275, -16.4782) -> (12.0401, -16.2575) ccw
  line L526 (12.1818, -13.8629) -> (12.053, -13.8703)
  line L527 (11.7968, -13.8892) -> (11.8891, -13.8839)
  line L528 (11.9656, -13.9107) -> (11.75, -13.9231)
  line L529 (11.8453, -13.749) -> (12.1615, -13.8599)
  line L530 (12.0327, -13.8673) -> (11.7757, -13.7772)
  line L531 (11.0496, -13.47) -> (11.3454, -13.5737)
  line L532 (11.4329, -13.7944) -> (11.3304, -15.8186)
  line L533 (11.224, -15.9714) -> (10.9282, -15.8676)
  line L534 (12.0401, -16.2575) -> (11.7239, -16.1466)
  line L535 (11.6364, -15.926) -> (11.7389, -13.9017)
  ellipse E418 centre (10.7061, -13.4897) end of major axis (11.1056, -13.5099) minor radius 0.0715 (11.0496, -13.47) -> (10.6167, -13.4156) ccw
  ellipse E419 centre (10.7061, -13.4897) end of major axis (10.4564, -13.4771) minor radius 0.0447 (10.9208, -13.4774) -> (10.7071, -13.445) ccw
  line L536 (11.2166, -13.5811) -> (10.9208, -13.4774)
  ellipse E420 centre (10.5847, -15.8874) end of major axis (10.1852, -15.8671) minor radius 0.0715 (10.9282, -15.8676) -> (10.4928, -15.8132) ccw
  line L537 (11.2016, -15.826) -> (11.3041, -13.8018)
  line L538 (9.8002, -15.612) -> (9.8157, -15.3065)
  line L539 (9.8774, -14.0875) -> (9.8992, -13.6572)
  line L540 (11.6791, -18.0306) -> (10.6484, -18.0898)
  line L541 (10.6468, -18.1211) -> (11.7556, -18.0574)
  ellipse E421 centre (11.6885, -17.8439) end of major axis (11.6257, -18.0232) minor radius 0.1599 (11.6791, -18.0306) -> (11.7695, -17.9954) ccw
  ellipse E422 centre (11.7651, -17.8707) end of major axis (11.7022, -18.05) minor radius 0.1599 (11.7556, -18.0574) -> (11.8531, -18.0164) ccw
  line L542 (12.2678, -13.7072) -> (12.3375, -12.3315)
  line L543 (12.25, -12.1108) -> (11.1382, -11.7209)
  line L544 (10.8396, -17.6167) -> (11.9515, -18.0066)
  line L545 (12.0579, -17.8539) -> (12.1275, -16.4782)
  line L546 (10.7108, -17.6241) -> (11.8227, -18.014)
  ellipse E423 centre (12.2406, -12.2975) end of major axis (12.2297, -12.1078) minor radius 0.0969 (12.3375, -12.3315) -> (12.25, -12.1108) ccw
  ellipse E424 centre (11.961, -17.8199) end of major axis (11.9719, -18.0096) minor radius 0.0969 (11.9515, -18.0066) -> (12.0579, -17.8539) ccw
  ellipse E425 centre (11.8322, -17.8273) end of major axis (11.8431, -18.017) minor radius 0.0969 (11.8227, -18.014) -> (11.8431, -18.017) ccw
  line L547 (11.9719, -18.0096) -> (11.8431, -18.017)
  ellipse E426 centre (11.336, -13.7604) end of major axis (11.3251, -13.5707) minor radius 0.0969 (11.4329, -13.7944) -> (11.3454, -13.5737) ccw
  ellipse E427 centre (11.2335, -15.7847) end of major axis (11.2444, -15.9744) minor radius 0.0969 (11.224, -15.9714) -> (11.3304, -15.8186) ccw
  ellipse E428 centre (11.7333, -15.9599) end of major axis (11.7442, -16.1496) minor radius 0.0969 (11.6364, -15.926) -> (11.7239, -16.1466) ccw
  ellipse E429 centre (11.8358, -13.9357) end of major axis (11.8249, -13.746) minor radius 0.0969 (11.8453, -13.749) -> (11.7389, -13.9017) ccw
  ellipse E430 centre (11.2072, -13.7678) end of major axis (11.1963, -13.5781) minor radius 0.0969 (11.3041, -13.8018) -> (11.2166, -13.5811) ccw
  ellipse E431 centre (10.1398, -13.6563) end of major axis (10.2027, -13.4771) minor radius 0.1599 (9.9804, -13.6349) -> (9.9786, -13.6454) ccw
  ellipse E432 centre (10.0633, -13.6295) end of major axis (10.0004, -13.8088) minor radius 0.1599 (9.9042, -13.6068) -> (9.9017, -13.6219) ccw
  ellipse E433 centre (9.9608, -15.6538) end of major axis (9.8979, -15.8331) minor radius 0.1599 (9.8024, -15.719) -> (9.8325, -15.7848) ccw
  ellipse E434 centre (10.0373, -15.6806) end of major axis (10.1002, -15.5013) minor radius 0.1599 (9.8766, -15.7341) -> (9.8906, -15.7805) ccw
  ellipse E435 centre (11.1047, -15.7921) end of major axis (11.1156, -15.9817) minor radius 0.0969 (11.1647, -15.9506) -> (11.2016, -15.826) ccw
  line L548 (9.6771, -17.6314) -> (10.3062, -17.5953)
  line L549 (10.2041, -17.57) -> (10.0036, -17.5815)
  line L550 (9.6531, -17.6016) -> (9.596, -17.6049)
  ellipse E436 centre (10.4961, -17.6365) end of major axis (10.7458, -17.6491) minor radius 0.0447 (10.7108, -17.6241) -> (10.5793, -17.5983) ccw
  ellipse E437 centre (10.7947, -11.7406) end of major axis (10.3952, -11.7204) minor radius 0.0715 (11.1382, -11.7209) -> (10.6513, -11.6668) ccw
  ellipse E438 centre (10.4961, -17.6365) end of major axis (10.0967, -17.6162) minor radius 0.0715 (10.8396, -17.6167) -> (10.4704, -17.5638) ccw
  ellipse E439 centre (-10.0315, -13.1918) end of major axis (-9.9732, -13.3726) minor radius 0.168 (-10.2017, -13.1796) -> (-10.0303, -13.3794) ccw
  ellipse E440 centre (-10.0983, -13.2133) end of major axis (-10.0399, -13.3941) minor radius 0.168 (-10.2281, -13.3242) -> (-10.0971, -13.401) ccw
  ellipse E441 centre (-10.0801, -15.9982) end of major axis (-10.1385, -15.8174) minor radius 0.168 (-10.1385, -15.8174) -> (-10.202, -15.8576) ccw
  ellipse E442 centre (-10.2871, -13.2068) end of major axis (-10.3007, -13.3963) minor radius 0.0836 (-10.2859, -13.3944) -> (-10.2026, -13.1795) ccw
  ellipse E443 centre (-10.4215, -13.1972) end of major axis (-10.4351, -13.3867) minor radius 0.0836 (-10.4202, -13.3848) -> (-10.3369, -13.1699) ccw
  ellipse E444 centre (-10.4033, -15.982) end of major axis (-10.3897, -15.7925) minor radius 0.0836 (-10.3188, -15.9547) -> (-10.4045, -15.7944) ccw
  ellipse E445 centre (-10.0134, -15.9766) end of major axis (-10.0718, -15.7958) minor radius 0.168 (-10.0146, -15.789) -> (-10.1836, -15.9644) ccw
  ellipse E446 centre (-10.269, -15.9917) end of major axis (-10.2554, -15.8022) minor radius 0.0836 (-10.1845, -15.9644) -> (-10.2554, -15.8022) ccw
  line L551 (-10.0718, -15.7958) -> (-10.1385, -15.8174)
  line L552 (-10.2554, -15.8022) -> (-10.3897, -15.7925)
  line L553 (-9.5964, -13.4369) -> (-10.0971, -13.401)
  line L554 (-10.0303, -13.3794) -> (-9.5297, -13.4153)
  line L555 (-10.696, -13.4739) -> (-10.6829, -13.4696)
  line L556 (-10.6815, -13.4692) -> (-10.4202, -13.3848)
  line L557 (-10.2859, -13.3944) -> (-10.4561, -13.4494)
  line L558 (-10.4045, -15.7944) -> (-10.5587, -15.8442)
  line L559 (-10.7661, -15.7231) -> (-10.7744, -14.4546)
  line L560 (-10.7772, -14.0133) -> (-10.7793, -13.6888)
  line L561 (-9.7576, -15.8075) -> (-10.0146, -15.789)
  line L562 (-10.645, -13.6984) -> (-10.6433, -13.9548)
  line L563 (-10.634, -15.3882) -> (-10.6318, -15.7328)
  ellipse E447 centre (-10.1073, -11.8308) end of major axis (-10.1657, -11.65) minor radius 0.168 (-10.1657, -11.65) -> (-10.2291, -11.6902) ccw